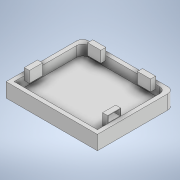
# Autodesk Inventor part: Lock
Saved by Autodesk Inventor 2021 (Build 250183000, 183)
## iProperties
Created: 2025-01-07
Part Number: Lock
Material: Generic
Document SubType Name: Modeling
Designer: 22liatho
Density: 1 g/cm^3
Appearance: Default
Author: 22liatho
Autodesk Inventor part; units mm, degrees
ref_plane "YZ Plane" through (0, 0, 0) normal (1, 0, 0) x (0, 1, 0)
ref_plane "XZ Plane" through (0, 0, 0) normal (0, 1, 0) x (-1, 0, 0)
sketch "Sketch1" plane through (0, 0, 0) normal (0, 1, 0) x (-1, 0, 0)
  line L0 (0, 0) -> (-45, 0)
  line L1 (-45, 0) -> (-45, -37.7)
  line L2 (-45, -37.7) -> (0, -37.7)
  line L3 (0, -37.7) -> (0, 0)
  dimension "d0" = 45
  dimension "d1" = 37.7
  constraints: 8 end point, 2 parallel, 1 horizontal, 1 perpendicular
  measures "d0" distance between parallel lines of L1 L3
  measures "d1" distance between parallel lines of L0 L2
extrude "Extrusion1" add sketch "Sketch1" along normal blind 2
sketch "Sketch2" plane through (0, 2, 0) normal (0, 1, 0) x (1, 0, 0)
  line L0 (2, 2) -> (43, 2)
  line L1 (43, 2) -> (43, 35.7)
  line L2 (43, 35.7) -> (2, 35.7)
  line L3 (2, 35.7) -> (2, 2)
  line L4 (0, 37.7) -> (0, 0) projected
  line L5 (45, 37.7) -> (0, 37.7) projected
  line L6 (45, 0) -> (45, 37.7) projected
  line L7 (0, 0) -> (45, 0) projected
  dimension "d4" = 2
  dimension "d5" = 2
  dimension "d6" = 2
  dimension "d7" = 2
  constraints: 8 end point, 2 parallel, 1 horizontal, 1 perpendicular
  measures "d4" distance between parallel lines of L6 L1
  measures "d5" distance between parallel lines of L5 L2
  measures "d6" distance between parallel lines of L4 L3
  measures "d7" distance between parallel lines of L7 L0
extrude "Extrusion2" add sketch "Sketch2" along normal blind 5
sketch "Sketch3" plane through (2, 2, -35.7) normal (0, 0, 1) x (1, 0, 0)
  line L0 (36, 3) -> (29.5, 3)
  line L1 (29.5, 3) -> (29.5, 8.5)
  line L2 (29.5, 8.5) -> (36, 8.5)
  line L3 (36, 8.5) -> (36, 3)
  line L4 (0, 5) -> (41, 5) projected
  line L5 (41, 0) -> (41, 5) projected
  point P0 (-2, -2)
  dimension "d10" = 3.5
  dimension "d11" = 6.5
  dimension "d12" = 5
  dimension "d13" = 2
  constraints: 8 end point, 2 parallel, 1 horizontal, 1 perpendicular
  measures "d10" distance between parallel lines of L4 L2
  measures "d11" distance between parallel lines of L1 L3
  measures "d12" distance between parallel lines of L5 L3
  measures "d13" distance between parallel lines of L4 L0
extrude "Extrusion3" add sketch "Sketch3" along normal blind 2.5
sketch "Sketch4" plane through (2, 2, -35.7) normal (0, 0, -1) x (-1, 0, 0)
  line L0 (-34.75, 7.25) -> (-30.75, 7.25)
  line L1 (-30.75, 7.25) -> (-30.75, 6.25)
  line L2 (-30.75, 6.25) -> (-34.75, 6.25)
  line L3 (-34.75, 6.25) -> (-34.75, 7.25)
  line L4 (-29.5, 8.5) -> (-29.5, 5) projected
  line L5 (-36, 8.5) -> (-29.5, 8.5) projected
  point P0 (2, -2)
  point P1 (-30.75, 6.75)
  point P2 (-29.5, 6.75)
  point P3 (-32.75, 7.25)
  point P4 (-32.75, 8.5)
  dimension "d16" = 1
  dimension "d17" = 4
  constraints: 8 end point, 4 midpoint, 2 parallel, 1 horizontal, 1 horizontal alignment, 1 perpendicular, 1 vertical alignment
  measures "d16" distance of L0.end L1.end
  measures "d17" distance of L0.start L0.end
extrude "Extrusion4" cut sketch "Sketch4" against normal blind 2
chamfer "Chamfer1" distance 1 distance2 2 1 edges at (32.75, 8.75, -35.7) measured on face at (35.4167, 7.4167, -35.7)
chamfer "Chamfer2" distance 1 distance2 2 1 edges at (36.75, 8.75, -35.7) measured on face at (35.4167, 7.4167, -35.7)
chamfer "Chamfer3" distance 1 distance2 2 1 edges at (34.75, 9.25, -35.7) measured on face at (35.4167, 7.4167, -35.7)
chamfer "Chamfer4" distance 1 distance2 2 1 edges at (34.75, 8.25, -35.7) measured on face at (35.4167, 7.4167, -35.7)
sketch "Sketch5" plane through (0, 0, 0) normal (0, -1, 0) x (1, 0, 0)
  line L0 (10, -27.7) -> (35, -27.7)
  line L1 (35, -27.7) -> (35, -10)
  line L2 (35, -10) -> (10, -10)
  line L3 (10, -10) -> (10, -27.7)
  line L4 (0, 0) -> (45, 0) projected
  line L5 (0, -37.7) -> (0, 0) projected
  line L6 (45, -37.7) -> (0, -37.7) projected
  line L7 (45, 0) -> (45, -37.7) projected
  dimension "d32" = 10
  dimension "d33" = 10
  dimension "d34" = 10
  dimension "d35" = 10
  constraints: 8 end point, 2 parallel, 1 horizontal, 1 perpendicular
  measures "d32" distance between parallel lines of L4 L2
  measures "d33" distance between parallel lines of L5 L3
  measures "d34" distance between parallel lines of L6 L0
  measures "d35" distance between parallel lines of L7 L1
extrude "Extrusion5" [suppressed]
sketch "Sketch7" plane through (43, 2, -35.7) normal (-1, 0, 0) x (0, 0, 1)
  line L0 (22.2, 3) -> (28.7, 3)
  line L1 (28.7, 3) -> (28.7, 8.5)
  line L2 (28.7, 8.5) -> (22.2, 8.5)
  line L3 (22.2, 8.5) -> (22.2, 3)
  line L4 (33.7, 0) -> (33.7, 5) projected
  line L5 (0, 5) -> (33.7, 5) projected
  point P0 (35.7, -2)
  dimension "d38" = 5
  dimension "d39" = 6.5
  dimension "d40" = 2
  dimension "d41" = 3.5
  constraints: 8 end point, 2 parallel, 1 horizontal, 1 perpendicular
  measures "d38" distance between parallel lines of L4 L1
  measures "d39" distance of L0.start L0.end
  measures "d40" distance between parallel lines of L5 L0
  measures "d41" distance between parallel lines of L5 L2
extrude "Extrusion6" add sketch "Sketch7" along normal blind 2.5
sketch "Sketch8" plane through (43, 2, -35.7) normal (1, 0, 0) x (0, 0, -1)
  line L0 (-27.45, 7.25) -> (-23.45, 7.25)
  line L1 (-23.45, 7.25) -> (-23.45, 6.25)
  line L2 (-23.45, 6.25) -> (-27.45, 6.25)
  line L3 (-27.45, 6.25) -> (-27.45, 7.25)
  line L4 (-22.2, 8.5) -> (-22.2, 5) projected
  line L5 (-22.2, 5) -> (-28.7, 5) projected
  point P0 (-35.7, -2)
  point P1 (-23.45, 6.75)
  point P2 (-22.2, 6.75)
  point P3 (-25.45, 5)
  point P4 (-25.45, 6.25)
  dimension "d44" = 4
  dimension "d45" = 1
  constraints: 8 end point, 4 midpoint, 2 parallel, 1 horizontal, 1 horizontal alignment, 1 perpendicular, 1 vertical alignment
  measures "d44" distance of L1.end L2.end
  measures "d45" distance of L0.end L1.end
extrude "Extrusion7" cut sketch "Sketch8" against normal blind 2
chamfer "Chamfer5" distance 1 distance2 2 1 edges at (43, 9.25, -10.25) measured on face at (43, 7.4167, -9.5833)
chamfer "Chamfer6" distance 1 distance2 2 1 edges at (43, 8.75, -8.25) measured on face at (43, 7.4167, -9.5833)
chamfer "Chamfer7" distance 1 distance2 2 1 edges at (43, 8.75, -12.25) measured on face at (43, 7.4167, -9.5833)
chamfer "Chamfer8" distance 1 distance2 2 1 edges at (43, 8.25, -10.25) measured on face at (43, 7.4167, -9.5833)
ref_plane "Work Plane1" through (22.5, 0, 0) normal (1, 0, 0) x (0, 0, -1)
mirror "Mirror1" about plane through (22.5, 0, 0) normal (1, 0, 0) of "Extrusion3", "Chamfer2", "Chamfer4", "Chamfer3", "Chamfer1", "Extrusion4"
mirror "Mirror2" about plane through (22.5, 0, 0) normal (1, 0, 0) of "Extrusion6", "Chamfer7", "Chamfer6", "Chamfer8", "Extrusion7", "Chamfer5"
fillet "Fillet1" radius 3 2 edges at (45, 3.5, -37.7) (0, 3.5, -37.7)
fillet "Fillet2" radius 3 2 edges at (2, 4.5, -35.7) (43, 4.5, -35.7)
body "Solid1"
